skadis_nut_right (Autodesk Fusion 360 design; units mm, degrees)
part number: 2026-09-06-14-40-23-923
Autodesk Fusion 360 part; units mm, degrees
sketch "Plate" plane through (0, 0, 0) normal (0, 1, 0) x (1, 0, 0)
  line L0 (0, 0) -> (11, 0)
  line L1 (11, 0) -> (11, -48)
  line L2 (11, -48) -> (0, -48)
  line L3 (0, -48) -> (0, 0)
  dimension "d359" = 11
  dimension "d360" = 48
  constraint coincident L0.start L3.end
  constraint horizontal L0
  constraint horizontal L2
  constraint vertical L1
  constraint vertical L3
  measures "d359" horizontal distance of L0.start L1.end
  measures "d360" vertical distance of L0.start L1.end
extrude "Plate (1)" add sketch "Plate" along normal mid plane 33 from surface at -4.5
sketch "Hook profile" plane through (0, 0, 0) normal (0, 1, 0) x (1, 0, 0)
  line L0 (0, -46) -> (-8.3, -46)
  line L1 (-8.3, -46) -> (-8.3, -29)
  line L2 (-8.3, -29) -> (-5.3, -29)
  line L3 (-5.3, -29) -> (-3.8, -30.5)
  line L4 (-3.8, -30.5) -> (-3.8, -41)
  line L5 (-3.8, -41) -> (0, -41)
  line L6 (0, -41) -> (0, -46)
  dimension "d364" = 46
  dimension "d365" = 8.3
  dimension "d366" = 3.8
  dimension "d367" = 5
  dimension "d368" = 10.5
  dimension "d369" = 1.5
  dimension "d370" = 1.5
  constraint horizontal L0
  constraint horizontal L2
  constraint horizontal L5
  constraint vertical L1
  constraint vertical L4
  constraint vertical L6
  constraint coincident origin L6
  measures "d364" vertical distance of origin L0.start
  measures "d365" horizontal distance of L0.start L0.end
  measures "d366" horizontal distance of L4.end L5.end
  measures "d367" vertical distance of L0.start L5.end
  measures "d368" vertical distance of L3.end L4.end
  measures "d369" horizontal distance of L2.end L3.end
  measures "d370" vertical distance of L2.end L3.end
extrude "Hook profile (1)" add sketch "Hook profile" along normal mid plane 2.4
pattern_linear "Hook rows" count 2 spacing 25.4 along (0, 0, -1) count 3 spacing 0 along (0, 0, 1) of "Hook profile (1)"
sketch "Screw hole" plane through (0, 0, 0) normal (0, 1, 0) x (1, 0, 0)
  line L0 (-1, -21.6) -> (12, -21.6)
  line L1 (12, -21.6) -> (12, -26.4)
  line L2 (12, -26.4) -> (-1, -26.4)
  line L3 (-1, -26.4) -> (-1, -21.6)
  dimension "d377" = 12
  dimension "d378" = 21.6
  dimension "d379" = 13
  dimension "d380" = 4.8
  constraint horizontal L0
  constraint horizontal L2
  constraint vertical L1
  constraint vertical L3
  measures "d377" horizontal distance of origin L0.end
  measures "d378" vertical distance of origin L0.end
  measures "d379" horizontal distance of L0.start L0.end
  measures "d380" vertical distance of L0.end L1.end
extrude "Screw hole (1)" cut sketch "Screw hole" along normal mid plane 16.8 from surface at -7.52
sketch "Nut cavity" plane through (0, 0, 0) normal (0, 1, 0) x (1, 0, 0)
  line L0 (3.6, -20.3) -> (7, -20.3)
  line L1 (7, -20.3) -> (7, -27.7)
  line L2 (7, -27.7) -> (3.6, -27.7)
  line L3 (3.6, -27.7) -> (3.6, -20.3)
  dimension "d384" = 7
  dimension "d385" = 20.3
  dimension "d386" = 3.4
  dimension "d387" = 7.4
  constraint horizontal L0
  constraint horizontal L2
  constraint vertical L1
  constraint vertical L3
  measures "d384" horizontal distance of origin L0.end
  measures "d385" vertical distance of origin L0.end
  measures "d386" horizontal distance of L0.start L0.end
  measures "d387" vertical distance of L0.end L1.end
extrude "Nut cavity (1)" cut sketch "Nut cavity" along normal mid plane 19.4 from surface at -7.52
sketch "Nut entry" plane through (0, 0, 0) normal (0, 1, 0) x (1, 0, 0)
  line L0 (3.6, -26.7) -> (7, -26.7)
  line L1 (7, -26.7) -> (7, -49)
  line L2 (7, -49) -> (3.6, -49)
  line L3 (3.6, -49) -> (3.6, -26.7)
  dimension "d391" = 7
  dimension "d392" = 26.7
  dimension "d393" = 3.4
  dimension "d394" = 22.3
  constraint horizontal L0
  constraint horizontal L2
  constraint vertical L1
  constraint vertical L3
  measures "d391" horizontal distance of origin L0.end
  measures "d392" vertical distance of origin L0.end
  measures "d393" horizontal distance of L0.start L0.end
  measures "d394" vertical distance of L0.end L1.end
extrude "Nut entry (1)" cut sketch "Nut entry" along normal mid plane 7.4 from surface at -1.52
sketch "Cavity roof" plane through (0, 0, 0) normal (0, 0, 1) x (1, 0, 0)
  line L0 (3.6, 2.18) -> (7, 2.18)
  line L1 (7, 2.18) -> (5.3, 3.88)
  line L2 (5.3, 3.88) -> (3.6, 2.18)
  dimension "d398" = 3.6
  dimension "d399" = 2.18
  dimension "d400" = 7
  dimension "d401" = 5.3
  dimension "d402" = 1.7
  constraint horizontal L0
  measures "d398" horizontal distance of origin L0.start
  measures "d399" vertical distance of origin L0.start
  measures "d400" horizontal distance of origin L0.end
  measures "d401" horizontal distance of origin L1.end
  measures "d402" vertical distance of L0.start L1.end
extrude "Cavity roof (1)" cut sketch "Cavity roof" along normal mid plane 29.7 from surface at 34.15
equation "bracketWidth = 24.0 mm" comment "bracket width across the upright"
equation "plateHeight = 48.0 mm" comment "plate height"
equation "plateInboardExtension = 9.0 mm" comment "extra plate toward the desk centre, where the channel reaches"
equation "boardThickness = 6.0 mm" comment "measured SKADIS panel thickness"
equation "screwLength = 15.0 mm" comment "measured decorative M4 screw"
equation "screwDiameter = 4.0 mm" comment "M4 shank"
equation "screwClearance = 0.8 mm" comment "slack around the shank"
equation "screwTipClearance = 2.0 mm" comment "tip stops this short of the plate's back face"
equation "screwSlotWidth = screwDiameter + screwClearance" comment "screw relief slot height"
equation "nutAcrossFlats = 7.0 mm" comment "M4 square nut across flats"
equation "nutThickness = 3.0 mm" comment "M4 square nut thickness"
equation "nutChannelClearance = 0.4 mm" comment "slack around the nut in its channel"
equation "nutChannelHeight = nutAcrossFlats + nutChannelClearance" comment "channel height; under the nut's diagonal so it cannot turn"
equation "plateThickness = screwLength - boardThickness + screwTipClearance" comment "derived: deep enough to swallow the screw"
equation "mountTravel = 12.0 mm" comment "left-right adjustment"
equation "nutChannelLength = mountTravel + nutAcrossFlats + nutChannelClearance" comment "channel length along the plate"
equation "screwSlotLength = mountTravel + screwSlotWidth" comment "relief slot length along the plate"
equation "topMountZ = 24.0 mm" comment "top channel centre"
equation "mountOffsetY = -7.52 mm" comment "channel centre on the board's grid"
equation "slotOvershoot = 1.0 mm" comment "cuts reach past the faces they cut"
equation "slotWidth = 3.2 mm" comment "measured upright slot width"
equation "slotPitchVertical = 25.4 mm" comment "1 inch, measured"
equation "faceMetalThickness = 2.0 mm" comment "upright face metal"
equation "hookTabWidth = slotWidth - 0.8 mm" comment "blade width through the slot"
equation "hookThroat = faceMetalThickness + 1.8 mm" comment "gap behind the plate"
equation "hookNeckHeight = 5.0 mm" comment "bears on the slot bottom edge"
equation "hookLipThickness = 4.5 mm" comment "lip behind the upright face"
equation "hookLipDrop = 12.0 mm" comment "engagement below the neck"
equation "hookLipChamfer = 1.5 mm" comment "lead-in past slot burrs"
equation "topHookNeckTop = plateHeight - 2 mm" comment "top hook row"
equation "hookRows = 2" comment "hook rows (pattern count)"
equation "nutCavityClearance = 0.4 mm" comment "slack across the nut's thickness"
equation "nutWallThickness = 4.0 mm" comment "wall in front of the nut; the screw pulls the nut against it"
equation "nutCavityDepth = nutThickness + nutCavityClearance" comment "cavity depth"
equation "nutRoofDepth = nutCavityDepth / 2" comment "45 deg roof beyond the cavity's outboard end, so it prints unsupported"
equation "d359 = plateThickness"
equation "d360 = plateHeight"
equation "d361 = -plateInboardExtension / 2"
equation "d362 = bracketWidth + plateInboardExtension"
equation "d364 = topHookNeckTop"
equation "d365 = hookThroat + hookLipThickness"
equation "d366 = hookThroat"
equation "d367 = hookNeckHeight"
equation "d368 = hookLipDrop - hookLipChamfer"
equation "d369 = hookLipChamfer"
equation "d370 = hookLipChamfer"
equation "d371 = hookTabWidth"
equation "d373 = hookRows"
equation "d375 = -slotPitchVertical"
equation "d377 = plateThickness + slotOvershoot"
equation "d378 = topMountZ - screwSlotWidth / 2"
equation "d379 = plateThickness + 2 * slotOvershoot"
equation "d380 = screwSlotWidth"
equation "d381 = mountOffsetY"
equation "d382 = screwSlotLength"
equation "d384 = plateThickness - nutWallThickness"
equation "d385 = topMountZ - nutChannelHeight / 2"
equation "d386 = nutCavityDepth"
equation "d387 = nutChannelHeight"
equation "d388 = mountOffsetY"
equation "d389 = nutChannelLength"
equation "d391 = plateThickness - nutWallThickness"
equation "d392 = topMountZ + nutChannelHeight / 2 - slotOvershoot"
equation "d393 = nutCavityDepth"
equation "d394 = plateHeight - topMountZ - nutChannelHeight / 2 + 2 * slotOvershoot"
equation "d395 = mountOffsetY + mountTravel / 2"
equation "d396 = nutChannelHeight"
equation "d398 = plateThickness - nutWallThickness - nutCavityDepth"
equation "d399 = mountOffsetY + nutChannelLength / 2"
equation "d400 = plateThickness - nutWallThickness"
equation "d401 = plateThickness - nutWallThickness - nutCavityDepth / 2"
equation "d402 = nutRoofDepth"
equation "d403 = ( topMountZ - nutChannelHeight / 2 + plateHeight ) / 2"
equation "d404 = plateHeight - topMountZ + nutChannelHeight / 2 + 2 * slotOvershoot"
named bodies: "skadis_nut_right"
